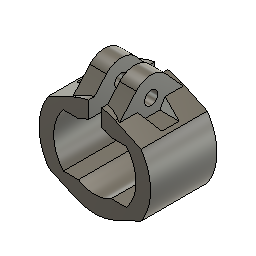
joint bracket v14 (Autodesk Fusion 360 design; units mm, degrees)
Autodesk Fusion 360 part; units mm, degrees
note: some values were not read from the file. Chosen so that the rebuilt part matches the saved one: which sketch regions a step uses.
sketch "Sketch1" plane through (0, 0, 0) normal (0, 0, 1) x (1, 0, 0)
  circle A0 centre (0, 0) radius 9.4
  circle A1 centre (0, 0) radius 12.4
  circle A2 centre (0, 0) radius 14.4
  line L0 (-14.3745, -7.7391) -> (14.9113, -7.7391)
  line L1 (-14.9113, 7.7391) -> (14.9113, 7.7391)
  circle A3 centre (0, 0) radius 16.8
  line L2 (0, 0) -> (0, -22) construction
  line L3 (0, 0) -> (0, 16.8) construction
  line L4 (-13.9241, -9.4) -> (-6.0799, -13.0535)
  line L5 (13.9241, -9.4) -> (6.0799, -13.0535)
  line L6 (-13.9241, 9.4) -> (-6.0799, 13.0535)
  line L7 (13.9241, 9.4) -> (6.0799, 13.0535)
  line L8 (-2, 0) -> (-2, 16.6805)
  line L9 (2, 0) -> (2, 16.6805)
  circle A4 centre (0, 0) radius 12.15
  line L10 (14.7788, -7.9891) -> (-14.7788, -7.9891)
  line L11 (-14.7788, 7.9891) -> (14.7788, 7.9891)
  line L12 (-13.9241, -9.4) -> (13.9241, -9.4) construction
  line L13 (-13.9241, 9.4) -> (13.9241, 9.4) construction
  dimension "PipeDiameter2" = 18.8
  dimension "d2" = 24.8
  dimension "d3" = 28.8
  dimension "d4" = 33.6
  dimension "d9" = 7.7391
  dimension "d10" = 7.7391
  dimension "d11" = 2
  dimension "d12" = 2
  dimension "d21" = 24.3
  dimension "d24" = 0.25
  dimension "d31" = 0.25
  measures "PipeDiameter2" diameter of A0
  measures "d2" diameter of A1
  measures "d3" diameter of A2
  measures "d4" diameter of A3
  measures "d9" distance of A0.centre L1
  measures "d10" distance of A0.centre L0
  measures "d11" distance of A0.centre L8
  measures "d12" distance of A0.centre L9
  measures "d21" diameter of A4
  measures "d24" distance of L0 L10
  measures "d31" distance of L1 L11
extrude "Extrude3" add sketch "Sketch1" along normal blind 20 contours A0 L9 A4 L11 | A0 A4 L10 | A1 L9 A4 L11 | A1 A2 L0 L1 | A1 A2 L1 L11 | A1 A4 L10 | A1 A2 L0 L10 | A0 L8 A4 L11 | A1 A2 L9 L11 | A2 L0 L1 A3 | A2 L1 A3 L11 | A1 A2 L10 | A1 A2 L0 L1 | A1 A2 L0 L10 | A2 L0 A3 L10 | A1 L8 A4 L11 | A2 A3 L7 L11 | A2 A3 L5 L10 | A1 A2 L1 L11 | A2 L1 A3 L10 | A1 A2 L8 L11 | A2 A3 L4 L10 | A2 L1 A3 L11 | A2 A3 L6 L11 makes body 1
sketch "Sketch2" plane through (0, 0, 0) normal (1, 0, 0) x (0, 0, -1)
  circle A0 centre (-10, 14.4) radius 2
  circle A1 centre (-10, 14.4) radius 6
  line L0 (-19.9458, 12.2207) -> (-14.4914, 18.3784)
  line L1 (0, 12.2207) -> (-5.5282, 18.4004)
  line L2 (0, 14.4) -> (0, -7.7391)
  line L3 (-19.9993, 9.1821) -> (-0.0276, 9.1821)
  line L4 (-20, 12) -> (-19.9993, 9.1821)
  line L5 (-4.8038, 14.3979) -> (-7.4001, 18.8989)
  line L6 (-7.4001, 18.8989) -> (-12.5962, 18.9011)
  line L7 (-12.5962, 18.9011) -> (-15.1962, 14.4021)
  line L8 (-15.1962, 14.4021) -> (-12.5999, 9.9011)
  line L9 (-12.5999, 9.9011) -> (-7.4038, 9.8989)
  line L10 (-7.4038, 9.8989) -> (-4.8038, 14.3979)
  line L11 (-20, 13.0535) -> (-20, 9.4)
  line L12 (-20, 9.1848) -> (-20, 14.2604)
  line L13 (-20, 9.4) -> (-20, 13.0535)
  line L14 (-20, 14.2604) -> (-20, 13.0535)
  line L15 (0, 12.2207) -> (-19.9458, 12.2207)
  dimension "d15" = 4
  dimension "d16" = 12
  dimension "d25" = 4.5
  dimension "d32" = 14.4
  measures "d15" diameter of A0
  measures "d16" diameter of A1
  measures "d25" distance of L10
  measures "d32" distance of origin
extrude "Extrude7" cut sketch "Sketch2" along normal mid plane 35 contours A0 | L5 L6 L7 L8 L10 L15 | L8 L9 L10 L15 bodies 1
extrude "Extrude8" add sketch "Sketch2" along normal mid plane 14 contours A1 L5 L6 L7 L8 L10 L15 | A1 L1 L15 | A1 L3 L8 L9 L10 L15 | A1 L0 L15 | L5 L6 L7 L8 L10 L15 | L8 L9 L10 L15 bodies 1
extrude "Extrude9" cut sketch "Sketch2" along normal mid plane 4 bodies 1
copy_body "Body->Comp2" bodies 1 removing the originals makes body 2 in component "joint bracket"
component "joint bracket" placed x (1, 0, 0) y (0, 1, 0) z (0, 0, 1) at (0, 0, 0)
equation "PipeDiameter2 = PipeDiameter + 1 mm"
equation "d2 = PipeDiameter2 + 6 mm"
equation "d3 = PipeDiameter2 + 10 mm"
equation "d4 = PipeDiameter + 15.8 mm"
equation "d9 = PipeDiameter / 2.3"
equation "d10 = PipeDiameter / 2.3"
equation "d11 = HalfOfScrewMount"
equation "d12 = HalfOfScrewMount"
equation "d15 = ScrewDiameter"
equation "d16 = ScrewDiameter * 3"
equation "d21 = d2 - Tolerance * 2"
equation "d24 = Tolerance"
equation "d25 = NutWidth / 2"
equation "PipeDiameter = 17.8 mm"
equation "Tolerance = 0.25 mm"
equation "HalfOfScrewMount = 2 mm"
equation "ScrewDiameter = 4 mm"
equation "NutWidth = 9 mm"
equation "d31 = Tolerance"
equation "d32 = ( PipeDiameter + 11 mm ) / 2"
